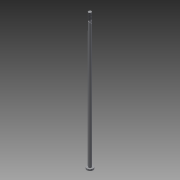
# Autodesk Inventor part: 19197 DSNU-12-200-P---(A---00--0-KS)
Saved by Autodesk Inventor 2014 SP2 (Build 180246200, 246)
## iProperties
Created: 2019-05-10
Part Number: 19197 DSNU-12-200-P---(A---00--0-KS)
Material: Generic
Catalog Web Link: www.cadenas.de
Description: DSNU---(KS)-Standard cylinder
Vendor: FESTO
Document SubType Name: Modeling
Designer: psadmin
Manufacturer: FESTO
Mass: 7.60965 g
Surface Area: 51.9975 cm^2
Volume: 7.60965 cm^3
Density: 1 g/cm^3
Appearance: PSOLRGB-192-192-192
Category: PARTsolutions
Company: FESTO
Title: 19197 DSNU-12-200-P
Author: Cadenas PARTsolutions
Comments: Standard cylinder
PSOL_IDENT_0: {$CADENAS_DATA\23d-libs\festo\parts\d\dsnu\parts\dsnu_metric_ks.prj},254 {VTYP=3D},{NB=19197 DSNU-12
PSOL_IDENT_1: -200-P---(A---00--0-KS)},{LINA=19197 DSNU-12-200-P},{NN=DSNU---(KS)},{DATE=21.02.2019 14:44:08},{GEO
PSOL_IDENT_2: MDATE=16.03.2016 12:59:00},{VERSION=},{LINEID=30},{WBVAR=TNR,HUB,DA,PE,ZD,VS,KA,K2A,K6,K3,K5,K8,KP},
PSOL_IDENT_3: {WBNUMERIC=HUB,K2A,K6,K8}  {NB=19197 DSNU-12-200-P---(A---00--0-KS)},{LINA=19197 DSNU-12-200-P},{KT=
PSOL_IDENT_4: DUMMY},{TNR=19197},{TYP=DSNU-12},{DSNU=METRIC},{KDM=12},{HUB=200},{DA=P},{DA1='P','PPV'},{PE=A},{ZD=
PSOL_IDENT_5: -},{VS=-},{VSALG='-','Q'},{KA=-},{KAALG='-','S2'},{K2A=0},{K6=0},{K3=-},{K31='-'},{K5=-},{K51='-'},{
PSOL_IDENT_6: K8=0},{KP=-},{KPALG='-','KP'},{A1=20},{A2=100},{A3=4},{A4=38.0},{AB=16},{AM=16},{B=16},{BB=3},{BE=M1
PSOL_IDENT_7: 6x1,5},{BENDM=16.000},{BEKDM=14.160},{BEP=1.500},{BS=4.5},{B1=30},{B2=0},{B3=0},{B4=0},{B5=18.1},{B6=
PSOL_IDENT_8: 8},{B7=0},{CD=6},{D=20},{D1=16},{D2=6},{D3=13.3},{D4=5.5},{D5=14.5},{D6=0},{D7=0},{EE=M5},{EENDM=5.0
PSOL_IDENT_9: 00},{EEKDM=4.019},{EW=12},{F=23},{FF=M4},{FFNDM=4.000},{FFKDM=3.141},{F1=0},{H=22},{H1=0},{KK=M6},{K
PSOL_IDENT_10: KNDM=6.000},{KKKDM=0.000},{KKP=1.000},{K1=-},{K1NDM=0.000},{K1KDM=0.000},{K2=0.0},{KV=24},{KW=8},{L=
PSOL_IDENT_11: 9},{LH=6.0},{LK=7.7},{L1=89},{L2=50},{L3=6.0},{L4=17.0},{L5=15},{L6=38},{L7=21},{L8=10.0},{L9=23.0},
PSOL_IDENT_12: {L10=61.8},{L11=71.8},{L12=47.7},{L13=94.0},{ST=4.5},{SW=5},{T=0},{WH=22},{X=0.0},{XC=75},{K1KP=32},
PSOL_IDENT_13: {K2KP=M5},{K2KPNDM=5.000},{K3KP=11},{K4KP=16.0},{K5KP=41.0},{K6KP=4.2},{K7KP=16},{K8KP=24.0},{K9KP=1
PSOL_IDENT_14: 0.0},{K10KP=0.0},{K11KP=0},{K12KP=M5},{K12KPNDM=5.000},{K13KP=38},{ZRSTART=27},{MHL=21.800},{ZRL=30}
PSOL_IDENT_15: ,{C=9.500},{WHX=10.000},{LD1=14.000},{LD2=13.700},{AD1=7.000},{AD2=5.000},{AD3=11.000},{AD4=6.000},{
PSOL_IDENT_16: AD5=0.000},{MH1=9.000},{MH2=3.200},{MH3=12.000},{KP1=22.500},{KP2=12.000},{KP3=9.600},{KP4=15.000},{
PSOL_IDENT_17: KP5=20.000},{KPC=14.000},{KPF=3.000},{KPG=10.000},{KPH=35.000},{KPJ=15.500},{KPK=11.000},{KPL=2.500}
PSOL_IDENT_18: ,{KPR3=0.800},{KPR=15.000},{KPS=8.500},{MLD1=30.000},{MLD2=24.000},{MLD3=4.000},{MLL1=10.000},{KL1=4
PSOL_IDENT_19: 2.3},{KKC=4.8},{KKD=1.5},{KKF=0.6},{SWL=3.000},{K3L=0.000},{HUB1=200},{FDTXF31=3.000},{FDTB31=3.200}
NN: DSNU---(KS)
NT: Standard cylinder
NB: 19197 DSNU-12-200-P---(A---00--0-KS)
NBSYN: $TNR. $TYP.-$HUB1.-$DA.---($PE.$ZD.$VS.$KA.$K2A.$K6.$K3.$K5.$K8.$KP.KS)
LINA: 19197 DSNU-12-200-P
TNR: 19197
TYP: DSNU-12
DSNU: METRIC
KDM: 12
HUB: 200
DA: P
DA1: 'P','PPV'
PE: A
ZD: -
VS: -
KA: -
K2A: 0
K6: 0
K3: -
K31: '-'
K5: -
K51: '-'
K8: 0
KP: -
A1: 20
A2: 100
A3: 4
A4: 38
AB: 16
AM: 16
B: 16
BB: 3
BE: M16x1,5
BENDM: 16
BEKDM: 14.16
BEP: 1.5
BS: 4.5
B1: 30
B2: 0
B3: 0
B4: 0
B5: 18.1
B6: 8
B7: 0
CD: 6
D: 20
D1: 16
D2: 6
D3: 13.3
D4: 5.5
D5: 14.5
D6: 0
D7: 0
EE: M5
EENDM: 5
EEKDM: 4.019
EW: 12
F: 23
FF: M4
FFNDM: 4
FFKDM: 3.141
F1: 0
H: 22
H1: 0
KK: M6
KKNDM: 6
KKKDM: 0
KKP: 1
K1: -
K1NDM: 0
K1KDM: 0
K2: 0
KV: 24
KW: 8
L: 9
LH: 6
LK: 7.7
L3: 6
L4: 17
L5: 15
L6: 38
L7: 21
L8: 10
L9: 23
L13: 94
ST: 4.5
SW: 5
T: 0
X: 0
K1KP: 32
K2KP: M5
K2KPNDM: 5
K3KP: 11
K4KP: 16
K5KP: 41
K6KP: 4.2
K7KP: 16
K8KP: 24
K9KP: 10
K10KP: 0
K11KP: 0
K12KP: M5
K12KPNDM: 5
K13KP: 38
MHL: 21.8
C: 9.5
WHX: 10
LD1: 14
LD2: 13.7
AD1: 7
AD2: 5
AD3: 11
AD4: 6
AD5: 0
MH1: 9
MH2: 3.2
MH3: 12
KP1: 22.5
KP2: 12
KP3: 9.6
KP4: 15
KP5: 20
KPC: 14
KPF: 3
KPG: 10
KPH: 35
KPJ: 15.5
KPK: 11
KPL: 2.5
KPR3: 0.8
KPR: 15
KPS: 8.5
MLD1: 30
MLD2: 24
MLD3: 4
MLL1: 10
SWL: 3
K3L: 0
FDTXF31: 3
FDTB31: 3.2
SUPPLIER: FESTO
ARTICLENO: 19197 DSNU-12-200-P---(A---00--0-KS)
BOMINFO: 19197 DSNU-12-200-P
CREATOR: CADENAS GmbH
Autodesk Inventor part; units mm, degrees
ref_plane "YZ Plane" through (0, 0, 0) normal (1, 0, 0) x (0, 1, 0)
ref_plane "XZ Plane" through (0, 0, 0) normal (0, 1, 0) x (-1, 0, 0)
ref_plane "XY Plane" through (0, 0, 0) normal (0, 0, 1) x (1, 0, 0)
sketch "Sketch_2" plane through (0, 0, 0) normal (1, 0, 0) x (0, 1, 0)
  line L0 (0, -240.3) -> (0, 5)
  line L1 (0, 5) -> (3, 5)
  line L2 (3, 5) -> (3, -237.3)
  line L3 (3, -237.3) -> (6, -237.3)
  line L4 (6, -237.3) -> (6, -240.3)
  line L5 (6, -240.3) -> (0, -240.3)
  line L6 (0, -240.3) -> (0, 5)
  constraints: 14 end point
revolve "Revolution1" add sketch "Sketch_2" angle 360 about axis through (0, 0, -240.3) along (0, 0, -1)
sketch "Sketch_6" plane through (0, 0, 0) normal (1, 0, 0) x (0, 1, 0)
  line L0 (0, 4) -> (0, 21)
  line L1 (0, 21) -> (2.3865, 21)
  line L2 (2.3865, 21) -> (3, 20.3865)
  line L3 (3, 20.3865) -> (3, 8.1485)
  line L4 (3, 8.1485) -> (2.4362, 6.5994)
  arc A0 (2.4362, 6.5994) -> (2.4, 6.3942) centre (3, 6.3942) ccw
  line L5 (2.4, 6.3942) -> (2.4, 5.6)
  arc A1 (2.4, 5.6) -> (3, 5) centre (3, 5.6) ccw
  line L6 (3, 5) -> (3, 4)
  line L7 (3, 4) -> (0, 4)
  line L8 (0, 4) -> (0, 21)
  constraints: 18 end point, 4 point on circle, 2 centre point
revolve "Revolution2" add sketch "Sketch_6" angle 360 about axis through (0, 0, 4) along (0, 0, -1)
thread "Thread1" size "M6x1" class "6g" standard "ISO Metric profile" full length
sketch "Sketch_7" plane through (0, 0, 2) normal (0, 0, 1) x (1, 0, 0)
  line L0 (-5, 10) -> (-5, -5)
  line L1 (-5, -5) -> (-2.5, -5)
  line L2 (-2.5, -5) -> (-2.5, 5)
  line L3 (-2.5, 5) -> (2.5, 5)
  line L4 (2.5, 5) -> (2.5, -5)
  line L5 (2.5, -5) -> (5, -5)
  line L6 (5, -5) -> (5, 10)
  line L7 (5, 10) -> (-5, 10)
  constraints: 16 end point
extrude "Extrusion1" cut sketch "Sketch_7" along normal blind 4
ref_plane "FDT_KSAUFSATZ_XY" through (0, 0, 11.2) normal (0, 0, 1) x (-1, 0, 0)
ref_plane "FDT_KSAUFSATZ_YZ" through (0, 0, 11.2) normal (-1, 0, 0) x (0, -1, 0)
ref_plane "FDT_KSAUFSATZ_ZX" through (0, 0, 11.2) normal (0, -1, 0) x (0, 0, 1)
ref_plane "FDT_NUT_XY" through (0, 0, 11.2) normal (0, 0, 1) x (-1, 0, 0)
ref_plane "FDT_NUT_YZ" through (0, 0, 11.2) normal (-1, 0, 0) x (0, -1, 0)
ref_plane "FDT_NUT_ZX" through (0, 0, 11.2) normal (0, -1, 0) x (0, 0, 1)
ref_plane "KS_XY" through (0, 0, 0) normal (0, 0, -1) x (1, 0, 0)
ref_plane "KS_YZ" through (0, 0, 0) normal (1, 0, 0) x (0, -1, 0)
ref_plane "KS_ZX" through (0, 0, 0) normal (0, -1, 0) x (0, 0, -1)
ref_plane "NUT1_XY" through (0, 0, 16) normal (0, 0, 1) x (1, 0, 0)
ref_plane "NUT1_YZ" through (0, 0, 16) normal (1, 0, 0) x (0, 1, 0)
ref_plane "NUT1_ZX" through (0, 0, 16) normal (0, 1, 0) x (0, 0, 1)
body "Solid1"
